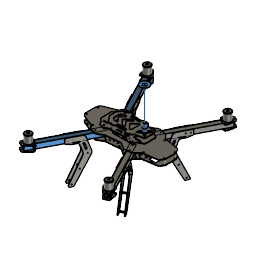
Arducopter (Autodesk Fusion 360 design; units mm, degrees)
Autodesk Fusion 360 part; units mm, degrees
note: some values were not read from the file. Chosen so that the rebuilt part matches the saved one: which bodies a step acts on; which face or edge a step refers to. Set by a fixed rule: which sketch regions a step uses.
(part 1 of 4)
other "Base Mesh Feature1"
sketch "Profile" plane through (0, 0, 0) normal (0, 0, 1) x (1, 0, 0) in component "Bottom Plate"
  line L0 (-165.6698, 0) -> (166.3965, 0) construction
  line L1 (-156, 0) -> (-156, 22.3832)
  line L2 (-155.0534, 25.3107) -> (-150.3466, 31.8278)
  line L3 (-148.1584, 33.5394) -> (-102.5293, 51.8851)
  line L4 (-100.1362, 53.9037) -> (-94.075, 63.7531)
  line L5 (-91.0078, 65.9886) -> (-68.4899, 71.5119)
  line L6 (-64.7398, 70.9514) -> (-43.9667, 58.5759)
  line L7 (-41.8797, 57.8938) -> (13.2682, 52.6642)
  line L8 (16.4597, 53.4461) -> (40.2244, 68.8491)
  line L9 (44.0623, 69.5267) -> (71.0992, 63.3215)
  line L10 (73.5163, 61.9837) -> (87.8503, 47.6497)
  line L11 (90.606, 46.2464) -> (143.7908, 37.8488)
  line L12 (147.2125, 35.6206) -> (155.2015, 23.2377)
  line L13 (156, 20.5271) -> (156, 0)
  arc A0 (-155.0534, 25.3107) -> (-156, 22.3832) centre (-151, 22.3832) ccw
  arc A1 (-148.1584, 33.5394) -> (-150.3466, 31.8278) centre (-146.2932, 28.9003) ccw
  arc A2 (-102.5293, 51.8851) -> (-100.1362, 53.9037) centre (-104.3945, 56.5242) ccw
  arc A3 (-91.0078, 65.9886) -> (-94.075, 63.7531) centre (-89.8167, 61.1326) ccw
  arc A4 (-64.7398, 70.9514) -> (-68.4899, 71.5119) centre (-67.2988, 66.6559) ccw
  arc A5 (-43.9667, 58.5759) -> (-41.8797, 57.8938) centre (-41.4077, 62.8714) ccw
  arc A6 (13.2682, 52.6642) -> (16.4597, 53.4461) centre (13.7403, 57.6419) ccw
  arc A7 (44.0623, 69.5267) -> (40.2244, 68.8491) centre (42.9439, 64.6534) ccw
  arc A8 (87.8503, 47.6497) -> (90.606, 46.2464) centre (91.3858, 51.1852) ccw
  arc A9 (73.5163, 61.9837) -> (71.0992, 63.3215) centre (69.9807, 58.4482) ccw
  arc A10 (147.2125, 35.6206) -> (143.7908, 37.8488) centre (143.011, 32.91) ccw
  arc A11 (156, 20.5271) -> (155.2015, 23.2377) centre (151, 20.5271) ccw
  circle A12 centre (-151.35, 22.65) radius 1.5
  circle A13 centre (-101.7, 47.55) radius 1.5
  circle A14 centre (-78.7284, 60.0301) radius 1.5
  circle A15 centre (-67, 37.5) radius 1.5
  circle A16 centre (44.5, 37.5) radius 1.5
  circle A17 centre (56.2284, 60.0301) radius 1.5
  circle A18 centre (90.7, 41.475) radius 1.5
  circle A19 centre (151.5, 21.3) radius 1.5
  line L14 (-51.5, 0) -> (-51.5, 8)
  line L15 (-48.5, 11) -> (-39, 11)
  line L16 (-36, 8) -> (-36, 0)
  arc A20 (-48.5, 11) -> (-51.5, 8) centre (-48.5, 8) ccw
  arc A21 (-36, 8) -> (-39, 11) centre (-39, 8) ccw
  line L17 (-24.5, 0) -> (-24.5, 8)
  arc A22 (-21.5, 11) -> (-24.5, 8) centre (-21.5, 8) ccw
  line L18 (-21.5, 11) -> (-12, 11)
  line L19 (-9, 8) -> (-9, 0)
  arc A23 (-9, 8) -> (-12, 11) centre (-12, 8) ccw
  line L20 (2.5, 0) -> (2.5, 8)
  arc A24 (5.5, 11) -> (2.5, 8) centre (5.5, 8) ccw
  line L21 (5.5, 11) -> (15, 11)
  line L22 (18, 8) -> (18, 0)
  arc A25 (18, 8) -> (15, 11) centre (15, 8) ccw
  line L23 (29.5, 0) -> (29.5, 8)
  arc A26 (32.5, 11) -> (29.5, 8) centre (32.5, 8) ccw
  line L24 (32.5, 11) -> (42, 11)
  line L25 (45, 8) -> (45, 0)
  arc A27 (45, 8) -> (42, 11) centre (42, 8) ccw
  line L26 (56.5, 0) -> (56.5, 8)
  arc A28 (59.5, 11) -> (56.5, 8) centre (59.5, 8) ccw
  line L27 (59.5, 11) -> (69, 11)
  line L28 (72, 8) -> (72, 0)
  arc A29 (72, 8) -> (69, 11) centre (69, 8) ccw
  line L29 (83.5, 0) -> (83.5, 8)
  arc A30 (86.5, 11) -> (83.5, 8) centre (86.5, 8) ccw
  line L30 (86.5, 11) -> (96, 11)
  line L31 (99, 8) -> (99, 0)
  arc A31 (99, 8) -> (96, 11) centre (96, 8) ccw
  line L32 (-138.8011, 33.9335) -> (-135.3218, 35.3324)
  line L33 (-137.9431, 31.7995) -> (-134.4638, 33.1984)
  line L34 (-111.0131, 45.106) -> (-107.5337, 46.5049)
  line L35 (-110.1551, 42.972) -> (-106.6758, 44.3709)
  arc A32 (-111.0131, 45.106) -> (-110.1551, 42.972) centre (-110.5841, 44.039) ccw
  arc A33 (-106.6758, 44.3709) -> (-107.5337, 46.5049) centre (-107.1047, 45.4379) ccw
  arc A34 (-138.8011, 33.9335) -> (-137.9431, 31.7995) centre (-138.3721, 32.8665) ccw
  arc A35 (-134.4638, 33.1984) -> (-135.3218, 35.3324) centre (-134.8928, 34.2654) ccw
  line L36 (-100.15, 23.25) -> (-78.65, 23.25)
  line L37 (-76.65, 21.25) -> (-76.65, 6.75)
  line L38 (-78.65, 4.75) -> (-100.15, 4.75)
  line L39 (-102.15, 6.75) -> (-102.15, 21.25)
  line L40 (-72.3, 26.65) -> (-67.8, 26.65)
  line L41 (-66.8, 25.65) -> (-66.8, 15.15)
  line L42 (-67.8, 14.15) -> (-72.3, 14.15)
  line L43 (-73.3, 15.15) -> (-73.3, 25.65)
  line L44 (-91.55, 29.2) -> (-88.6, 29.2)
  line L45 (-87.6, 28.2) -> (-87.6, 26.75)
  line L46 (-88.6, 25.75) -> (-91.55, 25.75)
  line L47 (-92.55, 26.75) -> (-92.55, 28.2)
  line L48 (-49, 33) -> (-23.5, 33)
  line L49 (-23.5, 30.25) -> (-49, 30.25)
  line L50 (-10.3083, 41.867) -> (-10.3083, 36.767)
  line L51 (-12.3083, 36.767) -> (-12.3083, 41.867)
  line L52 (0.1415, 48.7313) -> (5.2915, 48.7313)
  line L53 (5.2915, 46.2313) -> (0.1415, 46.2313)
  line L54 (0, 33.1) -> (28.75, 33.1)
  line L55 (28.75, 29.6) -> (0, 29.6)
  line L56 (69, 33.1) -> (94.75, 33.1)
  line L57 (94.75, 29.6) -> (69, 29.6)
  line L58 (105.8, 32.575) -> (127.3, 32.575)
  line L59 (129.3, 30.575) -> (129.3, 17.325)
  line L60 (127.3, 15.325) -> (105.8, 15.325)
  line L61 (103.8, 17.325) -> (103.8, 30.575)
  line L62 (114.175, 37.585) -> (118.925, 37.585)
  line L63 (118.925, 35.335) -> (114.175, 35.335)
  arc A36 (-136.5, 0) -> (-139.5, 0) centre (-138, 0) ccw
  arc A37 (-112.35, 0) -> (-115.35, 0) centre (-113.85, 0) ccw
  line L64 (-67, 37.5) -> (44.5, 37.5) construction
  line L65 (-67, 37.5) -> (-78.7284, 60.0301) construction
  line L66 (56.2284, 60.0301) -> (44.5, 37.5) construction
  line L67 (21.4122, 51.2935) -> (33.8182, 59.3344)
  line L68 (37.27, 55.2677) -> (25.061, 41.8506)
  line L69 (20.5, 43.6152) -> (20.5, 49.6152)
  arc A38 (37.27, 55.2677) -> (33.8182, 59.3344) centre (35.2809, 57.0777) ccw
  arc A39 (20.5, 43.6152) -> (25.061, 41.8506) centre (23.1219, 43.6152) ccw
  arc A40 (21.4122, 51.2935) -> (20.5, 49.6152) centre (22.5, 49.6152) ccw
  arc A41 (-100.15, 23.25) -> (-102.15, 21.25) centre (-100.15, 21.25) ccw
  arc A42 (-76.65, 21.25) -> (-78.65, 23.25) centre (-78.65, 21.25) ccw
  arc A43 (-78.65, 4.75) -> (-76.65, 6.75) centre (-78.65, 6.75) ccw
  arc A44 (-102.15, 6.75) -> (-100.15, 4.75) centre (-100.15, 6.75) ccw
  arc A45 (-72.3, 26.65) -> (-73.3, 25.65) centre (-72.3, 25.65) ccw
  arc A46 (-66.8, 25.65) -> (-67.8, 26.65) centre (-67.8, 25.65) ccw
  arc A47 (-67.8, 14.15) -> (-66.8, 15.15) centre (-67.8, 15.15) ccw
  arc A48 (-73.3, 15.15) -> (-72.3, 14.15) centre (-72.3, 15.15) ccw
  line L70 (-93.225, 0) -> (-93.225, 1)
  line L71 (-92.225, 2) -> (-87.925, 2)
  line L72 (-86.925, 1) -> (-86.925, 0)
  arc A49 (-92.225, 2) -> (-93.225, 1) centre (-92.225, 1) ccw
  arc A50 (-86.925, 1) -> (-87.925, 2) centre (-87.925, 1) ccw
  arc A51 (-91.55, 29.2) -> (-92.55, 28.2) centre (-91.55, 28.2) ccw
  arc A52 (-87.6, 28.2) -> (-88.6, 29.2) centre (-88.6, 28.2) ccw
  arc A53 (-88.6, 25.75) -> (-87.6, 26.75) centre (-88.6, 26.75) ccw
  arc A54 (-92.55, 26.75) -> (-91.55, 25.75) centre (-91.55, 26.75) ccw
  arc A55 (-49, 33) -> (-49, 30.25) centre (-49, 31.625) ccw
  arc A56 (-23.5, 30.25) -> (-23.5, 33) centre (-23.5, 31.625) ccw
  arc A57 (0, 33.1) -> (0, 29.6) centre (0, 31.35) ccw
  arc A58 (28.75, 29.6) -> (28.75, 33.1) centre (28.75, 31.35) ccw
  arc A59 (-10.3083, 41.867) -> (-12.3083, 41.867) centre (-11.3083, 41.867) ccw
  arc A60 (-12.3083, 36.767) -> (-10.3083, 36.767) centre (-11.3083, 36.767) ccw
  arc A61 (0.1415, 48.7313) -> (0.1415, 46.2313) centre (0.1415, 47.4813) ccw
  arc A62 (5.2915, 46.2313) -> (5.2915, 48.7313) centre (5.2915, 47.4813) ccw
  arc A63 (69, 33.1) -> (69, 29.6) centre (69, 31.35) ccw
  arc A64 (94.75, 29.6) -> (94.75, 33.1) centre (94.75, 31.35) ccw
  arc A65 (105.8, 32.575) -> (103.8, 30.575) centre (105.8, 30.575) ccw
  arc A66 (129.3, 30.575) -> (127.3, 32.575) centre (127.3, 30.575) ccw
  arc A67 (127.3, 15.325) -> (129.3, 17.325) centre (127.3, 17.325) ccw
  arc A68 (103.8, 17.325) -> (105.8, 15.325) centre (105.8, 17.325) ccw
  arc A69 (114.175, 37.585) -> (114.175, 35.335) centre (114.175, 36.46) ccw
  arc A70 (118.925, 35.335) -> (118.925, 37.585) centre (118.925, 36.46) ccw
  line L73 (103.8, 23.95) -> (129.3, 23.95) construction
  line L74 (116.55, 15.325) -> (116.55, 32.575) construction
  line L75 (116.55, 37.7058) -> (116.55, 35.335) construction
  line L76 (116.55, 10.1942) -> (116.55, 12.565) construction
  line L77 (118.925, 12.565) -> (114.175, 12.565)
  arc A71 (118.925, 10.315) -> (118.925, 12.565) centre (118.925, 11.44) ccw
  line L78 (114.175, 10.315) -> (118.925, 10.315)
  arc A72 (114.175, 12.565) -> (114.175, 10.315) centre (114.175, 11.44) ccw
  circle A73 centre (-55.4703, 45.1143) radius 2
  circle A74 centre (-37.4703, 45.1143) radius 2
  circle A75 centre (-46.4703, 52.1143) radius 2.5
  circle A76 centre (-46.4703, 38.1143) radius 2.5
  line L79 (-46.4703, 38.1143) -> (-46.4703, 52.1143) construction
  line L80 (-37.4703, 45.1143) -> (-55.4703, 45.1143) construction
  circle A77 centre (71.6389, 52.1143) radius 2.5
  circle A78 centre (71.6389, 38.1143) radius 2.5
  circle A79 centre (62.6389, 45.1143) radius 2
  circle A80 centre (80.6389, 45.1143) radius 2
  line L81 (62.6389, 45.1143) -> (80.6389, 45.1143) construction
  line L82 (71.6389, 52.1143) -> (71.6389, 38.1143) construction
  circle A81 centre (-25.7272, 40.0819) radius 2
  circle A82 centre (10.0728, 40.0819) radius 2
  line L83 (-25.7272, 40.0819) -> (10.0728, 40.0819) construction
  line L84 (0, -33.1) -> (28.75, -33.1)
  line L85 (0.1415, -48.7313) -> (5.2915, -48.7313)
  line L86 (-24.5, 0) -> (-24.5, -8)
  line L87 (-9, -8) -> (-9, 0)
  line L88 (-36, -8) -> (-36, 0)
  arc A83 (0, -29.6) -> (0, -33.1) centre (0, -31.35) ccw
  line L89 (28.75, -29.6) -> (0, -29.6)
  arc A84 (29.5, -8) -> (32.5, -11) centre (32.5, -8) ccw
  circle A85 centre (151.5, -21.3) radius 1.5
  arc A86 (25.061, -41.8506) -> (20.5, -43.6152) centre (23.1219, -43.6152) ccw
  line L90 (-72.3, -26.65) -> (-67.8, -26.65)
  arc A87 (94.75, -33.1) -> (94.75, -29.6) centre (94.75, -31.35) ccw
  line L91 (18, -8) -> (18, 0)
  circle A88 centre (71.6389, -38.1143) radius 2.5
  line L92 (-86.925, -1) -> (-86.925, 0)
  line L93 (-73.3, -15.15) -> (-73.3, -25.65)
  line L94 (116.55, -10.1942) -> (116.55, -12.565) construction
  line L95 (156, -20.5271) -> (156, 0)
  arc A89 (40.2244, -68.8491) -> (44.0623, -69.5267) centre (42.9439, -64.6534) ccw
  arc A90 (20.5, -49.6152) -> (21.4122, -51.2935) centre (22.5, -49.6152) ccw
  line L96 (-88.6, -25.75) -> (-91.55, -25.75)
  circle A91 centre (-46.4703, -38.1143) radius 2.5
  arc A92 (-72.3, -14.15) -> (-73.3, -15.15) centre (-72.3, -15.15) ccw
  line L97 (21.4122, -51.2935) -> (33.8182, -59.3344)
  line L98 (37.27, -55.2677) -> (25.061, -41.8506)
  line L99 (114.175, -37.585) -> (118.925, -37.585)
  circle A93 centre (62.6389, -45.1143) radius 2
  arc A94 (127.3, -32.575) -> (129.3, -30.575) centre (127.3, -30.575) ccw
  line L100 (103.8, -17.325) -> (103.8, -30.575)
  line L101 (16.4597, -53.4461) -> (40.2244, -68.8491)
  line L102 (-148.1584, -33.5394) -> (-102.5293, -51.8851)
  arc A95 (16.4597, -53.4461) -> (13.2682, -52.6642) centre (13.7403, -57.6419) ccw
  line L103 (-156, 0) -> (-156, -22.3832)
  arc A96 (-51.5, -8) -> (-48.5, -11) centre (-48.5, -8) ccw
  line L104 (-64.7398, -70.9514) -> (-43.9667, -58.5759)
  line L105 (2.5, 0) -> (2.5, -8)
  arc A97 (114.175, -10.315) -> (114.175, -12.565) centre (114.175, -11.44) ccw
  circle A98 centre (-67, -37.5) radius 1.5
  arc A99 (-110.1551, -42.972) -> (-111.0131, -45.106) centre (-110.5841, -44.039) ccw
  line L106 (-93.225, 0) -> (-93.225, -1)
  arc A100 (118.925, -12.565) -> (118.925, -10.315) centre (118.925, -11.44) ccw
  line L107 (56.2284, -60.0301) -> (44.5, -37.5) construction
  arc A101 (28.75, -33.1) -> (28.75, -29.6) centre (28.75, -31.35) ccw
  line L108 (-76.65, -21.25) -> (-76.65, -6.75)
  arc A102 (-68.4899, -71.5119) -> (-64.7398, -70.9514) centre (-67.2988, -66.6559) ccw
  line L109 (-46.4703, -38.1143) -> (-46.4703, -52.1143) construction
  line L110 (-100.1362, -53.9037) -> (-94.075, -63.7531)
  arc A103 (15, -11) -> (18, -8) centre (15, -8) ccw
  line L111 (118.925, -35.335) -> (114.175, -35.335)
  line L112 (5.5, -11) -> (15, -11)
  arc A104 (71.0992, -63.3215) -> (73.5163, -61.9837) centre (69.9807, -58.4482) ccw
  line L113 (71.6389, -52.1143) -> (71.6389, -38.1143) construction
  line L114 (-137.9431, -31.7995) -> (-134.4638, -33.1984)
  arc A105 (-66.8, -15.15) -> (-67.8, -14.15) centre (-67.8, -15.15) ccw
  circle A106 centre (-101.7, -47.55) radius 1.5
  line L115 (44.0623, -69.5267) -> (71.0992, -63.3215)
  arc A107 (-87.6, -26.75) -> (-88.6, -25.75) centre (-88.6, -26.75) ccw
  arc A108 (69, -11) -> (72, -8) centre (69, -8) ccw
  circle A109 centre (-151.35, -22.65) radius 1.5
  circle A110 centre (-55.4703, -45.1143) radius 2
  line L116 (72, -8) -> (72, 0)
  circle A111 centre (10.0728, -40.0819) radius 2
  line L117 (103.8, -23.95) -> (129.3, -23.95) construction
  arc A112 (-91.55, -25.75) -> (-92.55, -26.75) centre (-91.55, -26.75) ccw
  line L118 (-102.15, -6.75) -> (-102.15, -21.25)
  arc A113 (114.175, -35.335) -> (114.175, -37.585) centre (114.175, -36.46) ccw
  line L119 (-51.5, 0) -> (-51.5, -8)
  line L120 (116.55, -37.7058) -> (116.55, -35.335) construction
  line L121 (116.55, -15.325) -> (116.55, -32.575) construction
  line L122 (-67.8, -14.15) -> (-72.3, -14.15)
  arc A114 (-49, -30.25) -> (-49, -33) centre (-49, -31.625) ccw
  line L123 (-138.8011, -33.9335) -> (-135.3218, -35.3324)
  circle A115 centre (44.5, -37.5) radius 1.5
  arc A116 (2.5, -8) -> (5.5, -11) centre (5.5, -8) ccw
  arc A117 (-150.3466, -31.8278) -> (-148.1584, -33.5394) centre (-146.2932, -28.9003) ccw
  arc A118 (-73.3, -25.65) -> (-72.3, -26.65) centre (-72.3, -25.65) ccw
  arc A119 (-67.8, -26.65) -> (-66.8, -25.65) centre (-67.8, -25.65) ccw
  line L124 (90.606, -46.2464) -> (143.7908, -37.8488)
  arc A120 (5.2915, -48.7313) -> (5.2915, -46.2313) centre (5.2915, -47.4813) ccw
  line L125 (32.5, -11) -> (42, -11)
  line L126 (29.5, 0) -> (29.5, -8)
  circle A121 centre (-78.7284, -60.0301) radius 1.5
  line L127 (-111.0131, -45.106) -> (-107.5337, -46.5049)
  circle A122 centre (56.2284, -60.0301) radius 1.5
  arc A123 (69, -29.6) -> (69, -33.1) centre (69, -31.35) ccw
  line L128 (-110.1551, -42.972) -> (-106.6758, -44.3709)
  circle A124 centre (-46.4703, -52.1143) radius 2.5
  circle A125 centre (80.6389, -45.1143) radius 2
  arc A126 (-92.55, -28.2) -> (-91.55, -29.2) centre (-91.55, -28.2) ccw
  line L129 (114.175, -10.315) -> (118.925, -10.315)
  line L130 (86.5, -11) -> (96, -11)
  line L131 (-67, -37.5) -> (-78.7284, -60.0301) construction
  arc A127 (-93.225, -1) -> (-92.225, -2) centre (-92.225, -1) ccw
  line L132 (-66.8, -25.65) -> (-66.8, -15.15)
  arc A128 (90.606, -46.2464) -> (87.8503, -47.6497) centre (91.3858, -51.1852) ccw
  line L133 (59.5, -11) -> (69, -11)
  arc A129 (-135.3218, -35.3324) -> (-134.4638, -33.1984) centre (-134.8928, -34.2654) ccw
  arc A130 (-102.15, -21.25) -> (-100.15, -23.25) centre (-100.15, -21.25) ccw
  line L134 (118.925, -12.565) -> (114.175, -12.565)
  arc A131 (-156, -22.3832) -> (-155.0534, -25.3107) centre (-151, -22.3832) ccw
  line L135 (-92.55, -26.75) -> (-92.55, -28.2)
  arc A132 (103.8, -30.575) -> (105.8, -32.575) centre (105.8, -30.575) ccw
  arc A133 (42, -11) -> (45, -8) centre (42, -8) ccw
  line L136 (105.8, -32.575) -> (127.3, -32.575)
  arc A134 (-78.65, -23.25) -> (-76.65, -21.25) centre (-78.65, -21.25) ccw
  line L137 (127.3, -15.325) -> (105.8, -15.325)
  arc A135 (-41.8797, -57.8938) -> (-43.9667, -58.5759) centre (-41.4077, -62.8714) ccw
  arc A136 (56.5, -8) -> (59.5, -11) centre (59.5, -8) ccw
  arc A137 (-76.65, -6.75) -> (-78.65, -4.75) centre (-78.65, -6.75) ccw
  arc A138 (-115.35, 0) -> (-112.35, 0) centre (-113.85, 0) ccw
  arc A139 (129.3, -17.325) -> (127.3, -15.325) centre (127.3, -17.325) ccw
  arc A140 (-94.075, -63.7531) -> (-91.0078, -65.9886) centre (-89.8167, -61.1326) ccw
  arc A141 (105.8, -15.325) -> (103.8, -17.325) centre (105.8, -17.325) ccw
  arc A142 (-100.1362, -53.9037) -> (-102.5293, -51.8851) centre (-104.3945, -56.5242) ccw
  line L138 (-87.6, -28.2) -> (-87.6, -26.75)
  line L139 (-91.55, -29.2) -> (-88.6, -29.2)
  line L140 (99, -8) -> (99, 0)
  line L141 (-92.225, -2) -> (-87.925, -2)
  arc A143 (-88.6, -29.2) -> (-87.6, -28.2) centre (-88.6, -28.2) ccw
  circle A144 centre (90.7, -41.475) radius 1.5
  arc A145 (-137.9431, -31.7995) -> (-138.8011, -33.9335) centre (-138.3721, -32.8665) ccw
  arc A146 (143.7908, -37.8488) -> (147.2125, -35.6206) centre (143.011, -32.91) ccw
  arc A147 (155.2015, -23.2377) -> (156, -20.5271) centre (151, -20.5271) ccw
  line L142 (147.2125, -35.6206) -> (155.2015, -23.2377)
  arc A148 (96, -11) -> (99, -8) centre (96, -8) ccw
  line L143 (56.5, 0) -> (56.5, -8)
  arc A149 (83.5, -8) -> (86.5, -11) centre (86.5, -8) ccw
  line L144 (83.5, 0) -> (83.5, -8)
  arc A150 (-107.5337, -46.5049) -> (-106.6758, -44.3709) centre (-107.1047, -45.4379) ccw
  line L145 (-21.5, -11) -> (-12, -11)
  line L146 (-41.8797, -57.8938) -> (13.2682, -52.6642)
  circle A151 centre (-37.4703, -45.1143) radius 2
  line L147 (-67, -37.5) -> (44.5, -37.5) construction
  line L148 (-12.3083, -36.767) -> (-12.3083, -41.867)
  arc A152 (-10.3083, -36.767) -> (-12.3083, -36.767) centre (-11.3083, -36.767) ccw
  arc A153 (-12.3083, -41.867) -> (-10.3083, -41.867) centre (-11.3083, -41.867) ccw
  line L149 (-25.7272, -40.0819) -> (10.0728, -40.0819) construction
  line L150 (5.2915, -46.2313) -> (0.1415, -46.2313)
  line L151 (-10.3083, -41.867) -> (-10.3083, -36.767)
  line L152 (-100.15, -23.25) -> (-78.65, -23.25)
  line L153 (-78.65, -4.75) -> (-100.15, -4.75)
  line L154 (-155.0534, -25.3107) -> (-150.3466, -31.8278)
  arc A154 (0.1415, -46.2313) -> (0.1415, -48.7313) centre (0.1415, -47.4813) ccw
  arc A155 (-12, -11) -> (-9, -8) centre (-12, -8) ccw
  arc A156 (-23.5, -33) -> (-23.5, -30.25) centre (-23.5, -31.625) ccw
  line L155 (62.6389, -45.1143) -> (80.6389, -45.1143) construction
  line L156 (73.5163, -61.9837) -> (87.8503, -47.6497)
  line L157 (-91.0078, -65.9886) -> (-68.4899, -71.5119)
  arc A157 (-24.5, -8) -> (-21.5, -11) centre (-21.5, -8) ccw
  arc A158 (-39, -11) -> (-36, -8) centre (-39, -8) ccw
  line L158 (94.75, -29.6) -> (69, -29.6)
  circle A159 centre (-25.7272, -40.0819) radius 2
  line L159 (20.5, -43.6152) -> (20.5, -49.6152)
  arc A160 (-139.5, 0) -> (-136.5, 0) centre (-138, 0) ccw
  line L160 (-48.5, -11) -> (-39, -11)
  arc A161 (-100.15, -4.75) -> (-102.15, -6.75) centre (-100.15, -6.75) ccw
  arc A162 (33.8182, -59.3344) -> (37.27, -55.2677) centre (35.2809, -57.0777) ccw
  line L161 (-49, -33) -> (-23.5, -33)
  arc A163 (-87.925, -2) -> (-86.925, -1) centre (-87.925, -1) ccw
  arc A164 (118.925, -37.585) -> (118.925, -35.335) centre (118.925, -36.46) ccw
  line L162 (-37.4703, -45.1143) -> (-55.4703, -45.1143) construction
  circle A165 centre (71.6389, -52.1143) radius 2.5
  line L163 (-23.5, -30.25) -> (-49, -30.25)
  line L164 (69, -33.1) -> (94.75, -33.1)
  line L165 (45, -8) -> (45, 0)
  line L166 (129.3, -30.575) -> (129.3, -17.325)
  point P0 (-156, 24)
  point P1 (-149.5, 33)
  point P2 (-101, 52.5)
  point P3 (-93, 65.5)
  point P4 (-66.5, 72)
  point P5 (-43, 58)
  point P6 (15, 52.5)
  point P7 (42, 70)
  point P8 (72.5, 63)
  point P9 (89, 46.5)
  point P10 (146, 37.5)
  point P11 (156, 22)
  point P12 (-51.5, 11)
  point P13 (-36, 11)
  point P14 (-9, 11)
  point P15 (-24.5, 11)
  point P16 (18, 11)
  point P17 (2.5, 11)
  point P18 (45, 11)
  point P19 (29.5, 11)
  point P20 (72, 11)
  point P21 (56.5, 11)
  point P22 (99, 11)
  point P23 (83.5, 11)
  point P24 (-76.65, 23.25)
  point P25 (-76.65, 4.75)
  point P26 (-102.15, 4.75)
  point P27 (-92.55, 29.2)
  point P28 (-87.6, 29.2)
  point P29 (-87.6, 25.75)
  point P30 (129.3, 32.575)
  point P31 (129.3, 15.325)
  point P32 (103.8, 15.325)
  point P33 (-76.65, -4.75)
  point P34 (129.3, -15.325)
  point P35 (-24.5, -11)
  point P36 (99, -11)
  point P37 (-101, -52.5)
  point P38 (-87.6, -29.2)
  point P39 (89, -46.5)
  point P40 (72.5, -63)
  point P41 (146, -37.5)
  point P42 (103.8, -15.325)
  point P43 (72, -11)
  point P44 (156, -22)
  point P45 (-43, -58)
  point P46 (-87.6, -25.75)
  point P47 (-36, -11)
  point P48 (42, -70)
  point P49 (45, -11)
  point P50 (18, -11)
  point P51 (-149.5, -33)
  point P52 (-66.5, -72)
  point P53 (2.5, -11)
  point P54 (-9, -11)
  point P55 (-92.55, -29.2)
  point P56 (129.3, -32.575)
  point P57 (29.5, -11)
  point P58 (15, -52.5)
  point P59 (-76.65, -23.25)
  point P60 (83.5, -11)
  point P61 (-93, -65.5)
  point P62 (-51.5, -11)
  point P63 (56.5, -11)
  point P64 (-102.15, -4.75)
  dimension "d1" = 312
  dimension "d2" = 156
  dimension "d3" = 24
  dimension "d4" = 22
  dimension "d5" = 37.5
  dimension "d6" = 46.5
  dimension "d7" = 63
  dimension "d8" = 70
  dimension "d9" = 33
  dimension "d10" = 52.5
  dimension "d11" = 65.5
  dimension "d12" = 72
  dimension "d13" = 52.5
  dimension "d14" = 58
  dimension "d15" = 10
  dimension "d16" = 67
  dimension "d17" = 83.5
  dimension "d18" = 114
  dimension "d19" = 6.5
  dimension "d20" = 55
  dimension "d21" = 63
  dimension "d22" = 89.5
  dimension "d23" = 43
  dimension "d24" = 15
  dimension "d25" = 5
  dimension "d30" = 3
  dimension "d31" = 3
  dimension "d32" = 3
  dimension "d33" = 3
  dimension "d34" = 3
  dimension "d35" = 3
  dimension "d36" = 3
  dimension "d37" = 3
  dimension "d38" = 3
  dimension "d39" = 15.5
  dimension "d40" = 11
  dimension "d41" = 3
  dimension "d42" = 3
  dimension "d43" = 36
  dimension "d46" = 135
  dimension "d47" = 0
  dimension "d48" = 3.125
  dimension "d49" = 2.3
  dimension "d50" = 3.75
  dimension "d51" = 3.75
  dimension "d52" = 26.2
  dimension "d53" = 21.3
  dimension "d54" = 4.5
  dimension "d55" = 22.65
  dimension "d56" = 4.65
  dimension "d57" = 18
  dimension "d58" = 42.15
  dimension "d59" = 117.5
  dimension "d61" = 117.5
  dimension "d62" = 37.5
  dimension "d63" = 111.5
  dimension "d64" = 44.5
  dimension "d65" = 25.4
  dimension "d66" = 25.4
  dimension "d67" = 4.5
  dimension "d68" = 14.75
  dimension "d69" = 20.5
  dimension "d70" = 2
  dimension "d71" = 6
  dimension "d72" = 14.8
  dimension "d73" = 18.5
  dimension "d74" = 25.5
  dimension "d75" = 2
  dimension "d76" = 4.75
  dimension "d77" = 76.65
  dimension "d78" = 3.35
  dimension "d79" = 1
  dimension "d80" = 9.4
  dimension "d81" = 12.5
  dimension "d82" = 6.5
  dimension "d83" = 54.3
  dimension "d84" = 47.55
  dimension "d85" = 1
  dimension "d86" = 6.3
  dimension "d87" = 2
  dimension "d88" = 8.925
  dimension "d89" = 4.95
  dimension "d90" = 3.45
  dimension "d91" = 2.5
  dimension "d92" = 9.6
  dimension "d93" = 1
  dimension "d94" = 2.75
  dimension "d95" = 25.5
  dimension "d96" = 3.5
  dimension "d97" = 28.75
  dimension "d98" = 5.1
  dimension "d99" = 2
  dimension "d100" = 5.15
  dimension "d101" = 2.5
  dimension "d102" = 3.5
  dimension "d103" = 25.75
  dimension "d104" = 3
  dimension "d105" = 25.5
  dimension "d106" = 17.25
  dimension "d107" = 2
  dimension "d108" = 15.325
  dimension "d109" = 26.7
  dimension "d110" = 2.25
  dimension "d111" = 4.75
  dimension "d112" = 2.76
  dimension "d113" = 41.475
  dimension "d114" = 65.3
  dimension "d115" = 30.25
  dimension "d116" = 23.5
  dimension "d117" = 28.75
  dimension "d118" = 29.6
  dimension "d119" = 69
  dimension "d120" = 4
  dimension "d121" = 4
  dimension "d122" = 5
  dimension "d123" = 5
  dimension "d124" = 5
  dimension "d125" = 5
  dimension "d126" = 4
  dimension "d127" = 4
  dimension "d128" = 18
  dimension "d129" = 14
  dimension "d130" = 18
  dimension "d131" = 14
  dimension "d132" = 4
  dimension "d133" = 4
  dimension "d134" = 35.8
  constraint horizontal L0
  constraint coincident origin L0
  constraint coincident L0 L1.start
  constraint coincident L0 L13.end
  constraint vertical L1
  constraint vertical L13
  constraint coincident P0 L1
  constraint coincident P0 L2
  constraint tangent L1 A0
  constraint tangent L2 A0
  constraint coincident P1 L2
  constraint coincident P1 L3
  constraint tangent L2 A1
  constraint tangent L3 A1
  constraint equal A0 A1
  constraint coincident P2 L3
  constraint coincident P2 L4
  constraint tangent L3 A2
  constraint tangent L4 A2
  constraint equal A0 A2
  constraint coincident P3 L4
  constraint coincident P3 L5
  constraint tangent L4 A3
  constraint tangent L5 A3
  constraint equal A0 A3
  constraint coincident P4 L5
  constraint coincident P4 L6
  constraint tangent L5 A4
  constraint tangent L6 A4
  constraint equal A0 A4
  constraint coincident P5 L6
  constraint coincident P5 L7
  constraint tangent L6 A5
  constraint tangent L7 A5
  constraint equal A0 A5
  constraint coincident P6 L7
  constraint coincident P6 L8
  constraint tangent L7 A6
  constraint tangent L8 A6
  constraint equal A0 A6
  constraint coincident P7 L8
  constraint coincident P7 L9
  constraint tangent L8 A7
  constraint tangent L9 A7
  constraint equal A0 A7
  constraint coincident P9 L10
  constraint coincident P9 L11
  constraint tangent L10 A8
  constraint tangent L11 A8
  constraint equal A0 A8
  constraint coincident P8 L9
  constraint coincident P8 L10
  constraint tangent L9 A9
  constraint tangent L10 A9
  constraint equal A0 A9
  constraint coincident P10 L11
  constraint coincident P10 L12
  constraint tangent L11 A10
  constraint tangent L12 A10
  constraint equal A0 A10
  constraint coincident P11 L12
  constraint coincident P11 L13
  constraint tangent L12 A11
  constraint tangent L13 A11
  constraint equal A0 A11
  constraint coincident L0 A36.centre
  constraint coincident L0 A37.centre
  constraint coincident L0 L14.start
  constraint coincident L0 L16.end
  constraint coincident P12 L14
  constraint coincident P12 L15
  constraint tangent L14 A20
  constraint tangent L15 A20
  constraint coincident P13 L15
  constraint coincident P13 L16
  constraint tangent L15 A21
  constraint tangent L16 A21
  constraint vertical L16
  constraint horizontal L15
  constraint vertical L14
  constraint parallel L3 L32
  constraint parallel L32 L33
  constraint collinear L32 L34
  constraint collinear L33 L35
  constraint tangent L33 A34
  constraint tangent L32 A35
  constraint tangent L35 A32
  constraint tangent L34 A33
  constraint tangent L35 A33
  constraint tangent L34 A32
  constraint tangent L33 A35
  constraint tangent L32 A34
  constraint horizontal L36
  constraint vertical L37
  constraint horizontal L38
  constraint vertical L39
  constraint horizontal L40
  constraint vertical L41
  constraint horizontal L42
  constraint vertical L43
  constraint horizontal L44
  constraint vertical L45
  constraint horizontal L46
  constraint vertical L47
  constraint horizontal L48
  constraint horizontal L49
  constraint vertical L50
  constraint vertical L51
  constraint horizontal L52
  constraint horizontal L53
  constraint horizontal L54
  constraint horizontal L55
  constraint horizontal L56
  constraint horizontal L57
  constraint horizontal L58
  constraint vertical L59
  constraint horizontal L60
  constraint vertical L61
  constraint horizontal L62
  constraint horizontal L63
  constraint coincident L0 A36.end
  constraint coincident L0 A36.start
  constraint coincident L0 A37.end
  constraint coincident L0 A37.start
  constraint coincident A15.centre L64.start
  constraint coincident A16.centre L64.end
  constraint horizontal L64
  constraint coincident A14.centre L65.end
  constraint coincident A17.centre L66.start
  constraint parallel L8 L67
  constraint vertical L69
  constraint tangent L67 A38
  constraint tangent L68 A39
  constraint tangent L69 A39
  constraint tangent L68 A38
  constraint tangent L69 A40
  constraint tangent L67 A40
  constraint tangent L36 A41
  constraint tangent L39 A41
  constraint coincident P24 L36
  constraint coincident P24 L37
  constraint tangent L36 A42
  constraint tangent L37 A42
  constraint equal A41 A42
  constraint coincident P25 L37
  constraint coincident P25 L38
  constraint tangent L37 A43
  constraint tangent L38 A43
  constraint equal A41 A43
  constraint coincident P26 L38
  constraint coincident P26 L39
  constraint tangent L38 A44
  constraint tangent L39 A44
  constraint equal A41 A44
  constraint tangent L40 A45
  constraint tangent L43 A45
  constraint tangent L40 A46
  constraint tangent L41 A46
  constraint equal A45 A46
  constraint tangent L41 A47
  constraint tangent L42 A47
  constraint equal A45 A47
  constraint tangent L42 A48
  constraint tangent L43 A48
  constraint equal A45 A48
  constraint coincident L0 L70.start
  constraint coincident L0 L72.end
  constraint tangent L70 A49
  constraint tangent L71 A49
  constraint tangent L71 A50
  constraint tangent L72 A50
  constraint equal A49 A50
  constraint vertical L72
  constraint horizontal L71
  constraint vertical L70
  constraint coincident P27 L44
  constraint coincident P27 L47
  constraint tangent L44 A51
  constraint tangent L47 A51
  constraint coincident P28 L44
  constraint coincident P28 L45
  constraint tangent L44 A52
  constraint tangent L45 A52
  constraint equal A51 A52
  constraint coincident P29 L45
  constraint coincident P29 L46
  constraint tangent L45 A53
  constraint tangent L46 A53
  constraint equal A51 A53
  constraint tangent L46 A54
  constraint tangent L47 A54
  constraint equal A51 A54
  constraint tangent L49 A55
  constraint tangent L48 A56
  constraint tangent L48 A55
  constraint tangent L49 A56
  constraint tangent L55 A57
  constraint tangent L54 A58
  constraint tangent L55 A58
  constraint tangent L50 A59
  constraint tangent L51 A60
  constraint tangent L50 A60
  constraint tangent L51 A59
  constraint tangent L53 A62
  constraint tangent L53 A61
  constraint tangent L52 A62
  constraint tangent L52 A61
  constraint tangent L57 A63
  constraint tangent L57 A64
  constraint tangent L56 A63
  constraint tangent L56 A64
  constraint tangent L58 A65
  constraint tangent L61 A65
  constraint coincident P30 L58
  constraint coincident P30 L59
  constraint tangent L58 A66
  constraint tangent L59 A66
  constraint equal A65 A66
  constraint coincident P31 L59
  constraint coincident P31 L60
  constraint tangent L59 A67
  constraint tangent L60 A67
  constraint equal A65 A67
  constraint coincident P32 L60
  constraint coincident P32 L61
  constraint tangent L60 A68
  constraint tangent L61 A68
  constraint equal A65 A68
  constraint tangent L63 A70
  constraint tangent L63 A69
  constraint tangent L62 A69
  constraint tangent L62 A70
  constraint midpoint L61 L73.start
  constraint midpoint L59 L73.end
  constraint midpoint L60 L74.start
  constraint midpoint L58 L74.end
  constraint midpoint L63 L75.end
  constraint collinear L74 L75
  constraint symmetric L62.start L73 L78.start
  constraint symmetric L62.end L73 A71.start
  constraint symmetric L63.start L73 L77.start
  constraint symmetric L63.end L73 L77.end
  constraint symmetric A69 L73 A72
  constraint symmetric A70 L73 A71
  constraint symmetric L73 L75.start L76.start
  constraint symmetric L73 L75.end L76.end
  constraint collinear L54 L56
  constraint coincident A76.centre L79.start
  constraint coincident A75.centre L79.end
  constraint coincident A74.centre L80.start
  constraint coincident A73.centre L80.end
  constraint horizontal L80
  constraint vertical L79
  constraint midpoint L79 L80
  constraint coincident A79.centre L81.start
  constraint coincident A80.centre L81.end
  constraint coincident A77.centre L82.start
  constraint coincident A78.centre L82.end
  constraint horizontal L81
  constraint vertical L82
  constraint midpoint L81 L82
  constraint collinear L80 L81
  constraint coincident A81.centre L83.start
  constraint coincident A82.centre L83.end
  constraint horizontal L83
  constraint symmetric L0 L1.start L103.start
  constraint symmetric L0 P1 P51
  constraint symmetric L0 P2 P37
  constraint symmetric L0 P3 P61
  constraint symmetric L0 P4 P52
  constraint symmetric L0 P5 P45
  constraint symmetric L0 P6 P58
  constraint symmetric L0 P7 P48
  constraint symmetric L0 P8 P40
  constraint symmetric L0 P9 P39
  constraint symmetric L0 P10 P41
  constraint symmetric L0 P11 P44
  constraint symmetric L0 L13.end L95.end
  constraint symmetric L0 L1.end L103.end
  constraint symmetric L0 L2.start A131.end
  constraint symmetric L0 A0 A131
  constraint symmetric L0 L2.end A117.start
  constraint symmetric L0 L3.start L102.start
  constraint symmetric L0 A1 A117
  constraint symmetric L0 L3.end L102.end
  constraint symmetric L0 L4.start L110.start
  constraint symmetric L0 A2 A142
  constraint symmetric L0 L4.end L110.end
  constraint symmetric L0 L5.start A140.end
  constraint symmetric L0 A3 A140
  constraint symmetric L0 L5.end A102.start
  constraint symmetric L0 L6.start L104.start
  constraint symmetric L0 A4 A102
  constraint symmetric L0 L6.end L104.end
  constraint symmetric L0 L7.start A135.start
  constraint symmetric L0 A5 A135
  constraint symmetric L0 L7.end A95.end
  constraint symmetric L0 L8.start L101.start
  constraint symmetric L0 A6 A95
  constraint symmetric L0 L8.end A89.start
  constraint symmetric L0 L9.start A89.end
  constraint symmetric L0 A7 A89
  constraint symmetric L0 L10.end A128.end
  constraint symmetric L0 L11.start L124.start
  constraint symmetric L0 A8 A128
  constraint symmetric L0 L9.end A104.start
  constraint symmetric L0 L10.start A104.end
  constraint symmetric L0 A9 A104
  constraint symmetric L0 L11.end L124.end
  constraint symmetric L0 L12.start A146.end
  constraint symmetric L0 A10 A146
  constraint symmetric L0 L12.end A147.start
  constraint symmetric L0 L13.start L95.start
  constraint symmetric L0 A11 A147
  constraint symmetric L0 A12 A109
  constraint symmetric L0 A13 A106
  constraint symmetric L0 A14 A121
  constraint symmetric L0 A15 A98
  constraint symmetric L0 A16 A115
  constraint symmetric L0 A17 A122
  constraint symmetric L0 A18 A144
  constraint symmetric L0 A19 A85
  constraint symmetric L0 L14.start L119.start
  constraint symmetric L0 P12 P62
  constraint symmetric L0 P13 P47
  constraint symmetric L0 L16.end L88.end
  constraint symmetric L0 L14.end A96.start
  constraint symmetric L0 L15.start A96.end
  constraint symmetric L0 A20 A96
  constraint symmetric L0 L15.end A158.start
  constraint symmetric L0 L16.start L88.start
  constraint symmetric L0 A21 A158
  constraint symmetric L0 L17.start L86.start
  constraint symmetric L0 L17.end L86.end
  constraint symmetric L0 A22.start L145.start
  constraint symmetric L0 A22 A157
  constraint symmetric L0 P14 P54
  constraint symmetric L0 P15 P35
  constraint symmetric L0 L18.end L145.end
  constraint symmetric L0 L19.end L87.end
  constraint symmetric L0 L19.start L87.start
  constraint symmetric L0 A23 A155
  constraint symmetric L0 L20.start L105.start
  constraint symmetric L0 L20.end L105.end
  constraint symmetric L0 A24.start L112.start
  constraint symmetric L0 A24 A116
  constraint symmetric L0 P16 P50
  constraint symmetric L0 P17 P53
  constraint symmetric L0 L21.end A103.start
  constraint symmetric L0 L22.end L91.end
  constraint symmetric L0 L22.start L91.start
  constraint symmetric L0 A25 A103
  constraint symmetric L0 L23.start L126.start
  constraint symmetric L0 L23.end A84.start
  constraint symmetric L0 A26.start A84.end
  constraint symmetric L0 A26 A84
  constraint symmetric L0 P18 P49
  constraint symmetric L0 P19 P57
  constraint symmetric L0 L24.end L125.end
  constraint symmetric L0 L25.end L165.end
  constraint symmetric L0 L25.start A133.end
  constraint symmetric L0 A27 A133
  constraint symmetric L0 L26.start L143.start
  constraint symmetric L0 L26.end A136.start
  constraint symmetric L0 A28.start L133.start
  constraint symmetric L0 A28 A136
  constraint symmetric L0 P20 P43
  constraint symmetric L0 P21 P63
  constraint symmetric L0 L27.end A108.start
  constraint symmetric L0 L28.end L116.end
  constraint symmetric L0 L28.start A108.end
  constraint symmetric L0 A29 A108
  constraint symmetric L0 L29.start L144.start
  constraint symmetric L0 L29.end A149.start
  constraint symmetric L0 A30.start L130.start
  constraint symmetric L0 A30 A149
  constraint symmetric L0 P22 P36
  constraint symmetric L0 P23 P60
  constraint symmetric L0 L30.end L130.end
  constraint symmetric L0 L31.end L140.end
  constraint symmetric L0 L31.start L140.start
  constraint symmetric L0 A31 A148
  constraint symmetric L0 L32.start L123.start
  constraint symmetric L0 L32.end L123.end
  constraint symmetric L0 L33.start L114.start
  constraint symmetric L0 L33.end L114.end
  constraint symmetric L0 L34.start A99.end
  constraint symmetric L0 L34.end L127.end
  constraint symmetric L0 L35.start A99.start
  constraint symmetric L0 L35.end L128.end
  constraint symmetric L0 A32 A99
  constraint symmetric L0 A33 A150
  constraint symmetric L0 A34 A145
  constraint symmetric L0 A35 A129
  constraint symmetric L0 P24 P59
  constraint symmetric L0 P25 P33
  constraint symmetric L0 P26 P64
  constraint symmetric L0 P27 P55
  constraint symmetric L0 P28 P38
  constraint symmetric L0 P29 P46
  constraint symmetric L0 L48.start A114.end
  constraint symmetric L0 L48.end A156.start
  constraint symmetric L0 L49.start A156.end
  constraint symmetric L0 L49.end A114.start
  constraint symmetric L0 L51.end L148.end
  constraint symmetric L0 L50.start A153.end
  constraint symmetric L0 L50.end A152.start
  constraint symmetric L0 L51.start L148.start
  constraint symmetric L0 L52.start L85.start
  constraint symmetric L0 L52.end L85.end
  constraint symmetric L0 L53.start A120.end
  constraint symmetric L0 L53.end L150.end
  constraint symmetric L0 L54.start L84.start
  constraint symmetric L0 L54.end L84.end
  constraint symmetric L0 L55.start L89.start
  constraint symmetric L0 L55.end A83.start
  constraint symmetric L0 L56.start A123.end
  constraint symmetric L0 L56.end A87.start
  constraint symmetric L0 L57.start A87.end
  constraint symmetric L0 L57.end A123.start
  constraint symmetric L0 P30 P56
  constraint symmetric L0 P31 P34
  constraint symmetric L0 P32 P42
  constraint symmetric L0 L62.start L99.start
  constraint symmetric L0 L62.end L99.end
  constraint symmetric L0 L63.start L111.start
  constraint symmetric L0 L63.end L111.end
  constraint symmetric L0 A36.end A160.start
  constraint symmetric L0 A36.start A160.end
  constraint symmetric L0 A36 A160
  constraint symmetric L0 A37.end A138.start
  constraint symmetric L0 A37.start A138.end
  constraint symmetric L0 A37 A138
  constraint symmetric L0 A15.centre A98.centre
  constraint symmetric L0 A16.centre L107.end
  constraint symmetric L0 A14.centre A121.centre
  constraint symmetric L0 A17.centre L107.start
  constraint symmetric L0 L67.end L97.end
  constraint symmetric L0 L68.start L98.start
  constraint symmetric L0 L68.end A86.start
  constraint symmetric L0 L69.start A86.end
  constraint symmetric L0 A38 A162
  constraint symmetric L0 A39 A86
  constraint symmetric L0 L69.end A90.start
  constraint symmetric L0 L67.start A90.end
  constraint symmetric L0 A40 A90
  constraint symmetric L0 L36.start A130.end
  constraint symmetric L0 L39.end L118.end
  constraint symmetric L0 A41 A130
  constraint symmetric L0 L36.end A134.start
  constraint symmetric L0 L37.start L108.start
  constraint symmetric L0 A42 A134
  constraint symmetric L0 L37.end L108.end
  constraint symmetric L0 L38.start A137.end
  constraint symmetric L0 A43 A137
  constraint symmetric L0 L38.end L153.end
  constraint symmetric L0 L39.start L118.start
  constraint symmetric L0 A44 A161
  constraint symmetric L0 L40.start L90.start
  constraint symmetric L0 L43.end L93.end
  constraint symmetric L0 A45 A118
  constraint symmetric L0 L40.end L90.end
  constraint symmetric L0 L41.start A119.end
  constraint symmetric L0 A46 A119
  constraint symmetric L0 L41.end A105.start
  constraint symmetric L0 L42.start A105.end
  constraint symmetric L0 A47 A105
  constraint symmetric L0 L42.end A92.start
  constraint symmetric L0 L43.start L93.start
  constraint symmetric L0 A48 A92
  constraint symmetric L0 L70.start L106.start
  constraint symmetric L0 L72.end L92.end
  constraint symmetric L0 L70.end L106.end
  constraint symmetric L0 L71.start A127.end
  constraint symmetric L0 A49 A127
  constraint symmetric L0 L71.end L141.end
  constraint symmetric L0 L72.start L92.start
  constraint symmetric L0 A50 A163
  constraint symmetric L0 L44.start A126.end
  constraint symmetric L0 L47.end A126.start
  constraint symmetric L0 A51 A126
  constraint symmetric L0 L44.end L139.end
  constraint symmetric L0 L45.start L138.start
  constraint symmetric L0 A52 A143
  constraint symmetric L0 L45.end A107.start
  constraint symmetric L0 L46.start L96.start
  constraint symmetric L0 A53 A107
  constraint symmetric L0 L46.end L96.end
  constraint symmetric L0 L47.start A112.end
  constraint symmetric L0 A54 A112
  constraint symmetric L0 A55 A114
  constraint symmetric L0 A56 A156
  constraint symmetric L0 A57 A83
  constraint symmetric L0 A58 A101
  constraint symmetric L0 A59 A153
  constraint symmetric L0 A60 A152
  constraint symmetric L0 A61 A154
  constraint symmetric L0 A62 A120
  constraint symmetric L0 A63 A123
  constraint symmetric L0 A64 A87
  constraint symmetric L0 L58.start A132.end
  constraint symmetric L0 L61.end L100.end
  constraint symmetric L0 A65 A132
  constraint symmetric L0 L58.end A94.start
  constraint symmetric L0 L59.start A94.end
  constraint symmetric L0 A66 A94
  constraint symmetric L0 L59.end A139.start
  constraint symmetric L0 L60.start L137.start
  constraint symmetric L0 A67 A139
  constraint symmetric L0 L60.end L137.end
  constraint symmetric L0 L61.start L100.start
  constraint symmetric L0 A68 A141
  constraint symmetric L0 A69 A113
  constraint symmetric L0 A70 A164
  constraint symmetric L0 L73.start L117.start
  constraint symmetric L0 L73.end L117.end
  constraint symmetric L0 L74.start L121.start
  constraint symmetric L0 L74.end L121.end
  constraint symmetric L0 L75.start L120.start
  constraint symmetric L0 L75.end L120.end
  constraint symmetric L0 L77.start A100.start
  constraint symmetric L0 L77.end A97.end
  constraint symmetric L0 A71.start A100.end
  constraint symmetric L0 L78.start A97.start
  constraint symmetric L0 L76.end L94.end
  constraint symmetric L0 L76.start L94.start
  constraint symmetric L0 A71 A100
  constraint symmetric L0 A72 A97
  constraint symmetric L0 A73 A110
  constraint symmetric L0 A74 A151
  constraint symmetric L0 A75 A124
  constraint symmetric L0 A76 A91
  constraint symmetric L0 A76.centre A91.centre
  constraint symmetric L0 A75.centre L109.end
  constraint symmetric L0 A74.centre A151.centre
  constraint symmetric L0 A73.centre A110.centre
  constraint symmetric L0 A77 A165
  constraint symmetric L0 A78 A88
  constraint symmetric L0 A79 A93
  constraint symmetric L0 A80 A125
  constraint symmetric L0 A79.centre A93.centre
  constraint symmetric L0 A80.centre A125.centre
  constraint symmetric L0 A77.centre L113.start
  constraint symmetric L0 A78.centre A88.centre
  constraint symmetric L0 A81 A159
  constraint symmetric L0 A82 A111
  constraint symmetric L0 A81.centre L149.start
  constraint symmetric L0 A82.centre A111.centre
  measures "d1" distance of L1 L13
  measures "d2" distance of origin L13
  measures "d3" distance of L1.start P0
  measures "d4" distance of P11 L13.end
  measures "d5" distance of L0 P10
  measures "d6" distance of L0 P9
  measures "d7" distance of L0 P8
  measures "d8" distance of L0 P7
  measures "d9" distance of L0 P1
  measures "d10" distance of L0 P2
  measures "d11" distance of L0 P3
  measures "d12" distance of L0 P4
  measures "d13" distance of L0 P6
  measures "d14" vertical distance of origin P5
  measures "d15" distance of P10 L13
  measures "d16" distance of P9 L13
  measures "d17" distance of P8 L13
  measures "d18" distance of P7 L13
  measures "d19" distance of L1 P1
  measures "d20" distance of L1 P2
  measures "d21" distance of L1 P3
  measures "d22" distance of L1 P4
  measures "d23" horizontal distance of origin P5
  measures "d24" horizontal distance of origin P6
  measures "d25" radius of A0
  measures "d30" diameter of A12
  measures "d31" diameter of A36
  measures "d32" diameter of A37
  measures "d33" diameter of A13
  measures "d34" diameter of A14
  measures "d35" diameter of A15
  measures "d36" diameter of A16
  measures "d37" diameter of A17
  measures "d38" diameter of A19
  measures "d39" distance of P12 P13
  measures "d40" distance of P13 L16.end
  measures "d41" radius of A20
  measures "d42" radius of A21
  measures "d43" distance of origin L16
  measures "d48" distance of L3 L32
  measures "d49" distance of L32 L33
  measures "d50" distance of A32.centre A33.centre
  measures "d51" distance of A34.centre A35.centre
  measures "d52" distance of A35.centre A32.centre
  measures "d53" distance of L0 A19.centre
  measures "d54" distance of L13 A19.centre
  measures "d55" distance of L0 A12.centre
  measures "d56" distance of L1 A12.centre
  measures "d57" distance of L1 A36.centre
  measures "d58" distance of L1 A37.centre
  measures "d59" angle of L64 L66
  measures "d61" angle of L64 L65
  measures "d62" distance of L0 L64
  measures "d63" distance of A15.centre A16.centre
  measures "d64" horizontal distance of origin A16.centre
  measures "d65" distance of A17.centre A16.centre
  measures "d66" distance of A15.centre A14.centre
  measures "d67" distance of L8 L67
  measures "d68" angle of L67 L68
  measures "d69" distance of origin L69
  measures "d70" radius of A40
  measures "d71" vertical distance of A39.centre A40.centre
  measures "d72" distance of A38.centre A40.centre
  measures "d73" distance of P24 P25
  measures "d74" distance of P25 P26
  measures "d75" radius of A41
  measures "d76" distance of L0 L38
  measures "d77" distance of origin L37
  measures "d78" distance of L37 L43
  measures "d79" radius of A45
  measures "d80" distance of L38 L42
  measures "d81" distance of L40 L42
  measures "d82" distance of L41 L43
  measures "d83" distance of L1 A13.centre
  measures "d84" distance of L0 A13.centre
  measures "d85" radius of A49
  measures "d86" distance of L70 L72
  measures "d87" distance of L0 L71
  measures "d88" distance of L39 L70
  measures "d89" distance of P27 P28
  measures "d90" distance of P28 P29
  measures "d91" distance of L36 L46
  measures "d92" distance of L39 L47
  measures "d93" radius of A51
  measures "d94" distance of L48.start L49.end
  measures "d95" distance of A55.centre A56.centre
  measures "d96" distance of L54.start L55.end
  measures "d97" distance of A57.centre A58.centre
  measures "d98" distance of A59.centre A60.centre
  measures "d99" distance of L50 L51
  measures "d100" distance of A62.centre A61.centre
  measures "d101" distance of L52 L53
  measures "d102" distance of L56 L57
  measures "d103" distance of A63.centre A64.centre
  measures "d104" diameter of A18
  measures "d105" distance of P31 P32
  measures "d106" distance of P30 P31
  measures "d107" radius of A65
  measures "d108" distance of L0 L60
  measures "d109" distance of L13 L59
  measures "d110" distance of L62 L63
  measures "d111" distance of A70.centre A69.centre
  measures "d112" distance of L58 L63
  measures "d113" distance of L0 A18.centre
  measures "d114" distance of L13 A18.centre
  measures "d115" distance of L0 L49
  measures "d116" horizontal distance of origin A56.centre
  measures "d117" horizontal distance of origin A58.centre
  measures "d118" distance of L0 L55
  measures "d119" horizontal distance of origin A63.centre
  measures "d120" diameter of A73
  measures "d121" diameter of A74
  measures "d122" diameter of A75
  measures "d123" diameter of A76
  measures "d124" diameter of A77
  measures "d125" diameter of A78
  measures "d126" diameter of A79
  measures "d127" diameter of A80
  measures "d128" distance of A79.centre A80.centre
  measures "d129" distance of A77.centre A78.centre
  measures "d130" distance of A74.centre A73.centre
  measures "d131" distance of A76.centre A75.centre
  measures "d132" diameter of A81
  measures "d133" diameter of A82
  measures "d134" distance of A81.centre A82.centre
extrude "Extrude1" add sketch "Profile" along normal blind 2 makes body 1 in component "Bottom Plate"